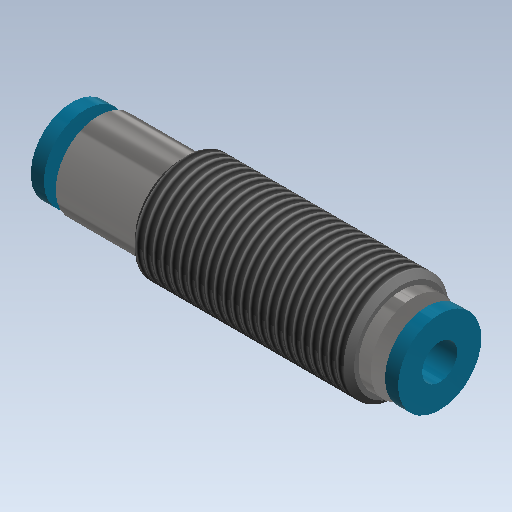
# Autodesk Inventor part: KCE04-00(5-3)_BU_BODY
Saved by Autodesk Inventor 2021 (Build 250183000, 183)
## iProperties
Part Number: KCE04-00(5-3)_BU_BODY
Material: Generic
Catalog Web Link: www.cadenas.de
Description: KCE BU BODY-Bulkhead Union
Vendor: SMC
Document SubType Name: Modeling
Designer: partserver
Manufacturer: SMC
Mass: 21 g
Surface Area: 22.4886 cm^2
Volume: 3.49152 cm^3
Density: 1 g/cm^3
Appearance: PSOLRGB-128-128-128
Category: PARTsolutions
Company: SMC
PSOL_IDENT_0: {$CADENAS_DATA\23d-libs\smc_jp\fittings_and_tubing\fittings_for_general_purposes\kc\kce_bu\parts\kce
PSOL_IDENT_1: _bu_body.prj},196 {VTYP=3D},{NB=KCE04-00(5-3)_BU_BODY},{LINA=KCE04-00_BU_BODY},{NN=KCE BU BODY},{DAT
PSOL_IDENT_2: E=30.01.2020 13:12:38},{GEOMDATE=17.10.2018 06:50:00},{VERSION=},{LINEID=10},{WBVAR=MPT,POS},{WBNUME
PSOL_IDENT_3: RIC=MPT,POS}  {NB=KCE04-00(5-3)_BU_BODY},{LINA=KCE04-00_BU_BODY},{KT=DUMMY},{OD=4},{MODEL=KCE04-00},
PSOL_IDENT_4: {MPT=5},{POS=3},{T=M12x1},{RA=12},{RP=1},{L=42.0},{LH1=1.5},{LH2=1.5},{LH3=1.4},{LH4=5.0},{LH5=25.1}
PSOL_IDENT_5: ,{DV1=5.0},{DV2=9.5},{DV3=9.8},{DV4=0},{MH=13},{M1=18.0},{M2=16.0},{EA1=2.6},{EA2=2.6},{CNSMASSEXACT=
PSOL_IDENT_6: 21},{NENN=KCE04-00},{MAX=10.1}
NB: KCE04-00(5-3)_BU_BODY
NN: KCE BU BODY
NT: Bulkhead Union
NBSYN: $MODEL.($MPT.-$POS.)_BU_BODY
LINA: KCE04-00_BU_BODY
CATALOG: SMC (JP
OD: 4
MODEL: KCE04-00
MPT: 5
POS: 3
T: M12x1
RA: 12
RP: 1
L: 42
MH: 13
M1: 18
M2: 16
EA1: 2.6
EA2: 2.6
CNSMASSEXACT: 21
SUPPLIER: SMC
ARTICLENO: KCE04-00(5-3)_BU_BODY
BOMINFO: KCE04-00_BU_BODY
CREATOR: CADENAS GmbH
Title: KCE04-00_BU_BODY
Author: Cadenas PARTsolutions
Comments: Bulkhead Union
Autodesk Inventor part; units mm, degrees
sketch "Sketch_1" plane through (0, 0, 0) normal (0, 0, 1) x (1, 0, 0)
  line L0 (42, 0) -> (0, 0)
  line L1 (16, 0) -> (16, 2)
  line L2 (16, 2) -> (0, 2)
  line L3 (0, 2) -> (0, 4.75)
  line L4 (0, 4.75) -> (1.5, 4.75)
  line L5 (1.5, 4.75) -> (1.5, 2.5)
  line L6 (1.5, 2.5) -> (3, 2.5)
  line L7 (3, 2.5) -> (3, 4.9)
  line L8 (3, 4.9) -> (4.4, 4.9)
  line L9 (4.4, 4.9) -> (4.4, 5.3865)
  line L10 (4.4, 5.3865) -> (5.0135, 6)
  line L11 (5.0135, 6) -> (28.8865, 6)
  line L12 (28.8865, 6) -> (29.5, 5.3865)
  line L13 (29.5, 5.3865) -> (29.5, 4.9)
  line L14 (29.5, 4.9) -> (39, 4.9)
  line L15 (39, 4.9) -> (39, 2.5)
  line L16 (39, 2.5) -> (40.5, 2.5)
  line L17 (40.5, 2.5) -> (40.5, 4.75)
  line L18 (40.5, 4.75) -> (42, 4.75)
  line L19 (42, 4.75) -> (42, 2)
  line L20 (42, 2) -> (24, 2)
  line L21 (24, 2) -> (24, 0)
  line L22 (24, 0) -> (16, 0)
  constraints: 46 end point
revolve "Revolution1" add sketch "Sketch_1" angle 360 about axis through (42, 0, 0) along (1, 0, 0)
thread "Thread1" size "M12x1" class "6g" standard "ISO Metric profile" full length
ref_plane "IP1_XY" through (0, 0, 0) normal (1, 0, 0) x (0, 0, -1)
ref_plane "IP1_YZ" through (0, 0, 0) normal (0, 0, -1) x (0, 1, 0)
ref_plane "IP1_ZX" through (0, 0, 0) normal (0, 1, 0) x (1, 0, 0)
ref_plane "IP2_XY" through (7.4, 0, 0) normal (-1, 0, 0) x (0, 0, -1)
ref_plane "IP2_YZ" through (7.4, 0, 0) normal (0, 0, -1) x (0, -1, 0)
ref_plane "IP2_ZX" through (7.4, 0, 0) normal (0, -1, 0) x (-1, 0, 0)
ref_plane "IP3_XY" through (17.4, 0, 0) normal (-1, 0, 0) x (0, 0, -1)
ref_plane "IP3_YZ" through (17.4, 0, 0) normal (0, 0, -1) x (0, -1, 0)
ref_plane "IP3_ZX" through (17.4, 0, 0) normal (0, -1, 0) x (-1, 0, 0)
body "Solid1"
